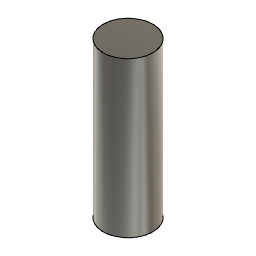
Lymphedema Project  Assembly v12 (Autodesk Fusion 360 archive; units mm, degrees)
design "Hand Model"
Autodesk Fusion 360 part; units mm, degrees
sketch "Sketch1" plane through (0, 0, 0) normal (0, 1, 0) x (1, 0, 0)
  circle A0 through (40, 0, 0) (-20, 0, 34.641) (-20, 0, -34.641)
  dimension "d1" = 80
extrude "Extrude1" add sketch "Sketch1" against normal blind 250 contours A0 in plane through (0, 0, 0) normal (0, 0, -1)

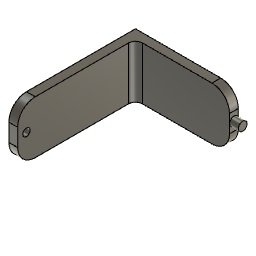
design "dummy wheel bracket"
Autodesk Fusion 360 part; units mm, degrees
sketch "Sketch1" plane through (0, 0, 0) normal (0, 0, 1) x (1, 0, 0)
  line L0 (-50, 0) -> (3.5, 0)
  line L1 (-50, 0) -> (-50, -67)
  line L2 (-50, -67) -> (-55, -67)
  line L3 (-55, -67) -> (-55, 5)
  line L4 (-55, 5) -> (3.5, 5)
  line L5 (3.5, 5) -> (3.5, 0)
  dimension "d1" = 53.5
  dimension "d2" = 67
  dimension "d3" = 5
  dimension "d8" = 5
  constraint horizontal L0
  constraint perpendicular L0 L1
  constraint perpendicular L1 L2
  constraint perpendicular L2 L3
  constraint perpendicular L3 L4
  measures "d1" distance of L0.start L0.end
  measures "d2" distance of L0.start L1.end
  measures "d3" distance of L1.end L2.end
  measures "d8" distance of L0.end L4.end
extrude "Extrude1" add sketch "Sketch1" along normal blind 30
sketch "Sketch2" plane through (3.5, 0, 0) normal (1, 0, 0) x (0, 1, 0)
  line L0 (0, 0) -> (5, 0)
  line L1 (5, 0) -> (5, 30)
  line L2 (5, 30) -> (0, 30)
  line L3 (0, 30) -> (0, 0)
  circle A0 centre (2.5, 15) radius 2.5
  dimension "d10" = 5
  measures "d10" diameter of A0
extrude "Extrude2" add sketch "Sketch2" along normal blind 5 contours A0
sketch "Sketch3" plane through (-50, 0, 0) normal (1, 0, 0) x (0, 1, 0)
  line L0 (-67, 0) -> (0, 0)
  line L1 (0, 0) -> (0, 30)
  line L2 (0, 30) -> (-67, 30)
  line L3 (-67, 30) -> (-67, 0)
  circle A0 centre (-62, 15) radius 2.1
  dimension "d14" = 4.2
  dimension "d17" = 5
  measures "d14" diameter of A0
  measures "d17" distance of L3 A0.centre
extrude "Extrude3" cut sketch "Sketch3" against normal blind 12 contours A0
fillet "Fillet1" radius 10 4 edges at (-52.5, -67, 30) (-52.5, -67, 0) (3.5, 2.5, 0) (3.5, 2.5, 30)
fillet "Fillet2" radius 4 1 edges at (-50, 0, 15)
equation "d1 = ( 117 / 2 ) * 1 mm - 5 mm"
equation "d2 = 100 mm - 33 mm"

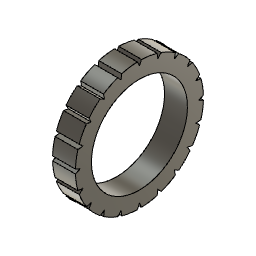
design "Soft Robotic Silicone Ring"
Autodesk Fusion 360 part; units mm, degrees
sketch "Sketch1" plane through (0, 0, 0) normal (0, 0, 1) x (1, 0, 0)
  line L0 (0, -42) -> (-10, -42)
  line L1 (-10, -42) -> (-10, -56)
  line L2 (-10, -56) -> (10, -56)
  line L3 (10, -56) -> (10, -42)
  line L4 (10, -42) -> (0, -42)
  dimension "d1" = 42
  dimension "d2" = 10
  dimension "d3" = 14
  dimension "d4" = 20
  dimension "d5" = 14
  constraint perpendicular L0 L1
  constraint perpendicular L1 L2
  constraint perpendicular L2 L3
  measures "d1" distance of origin L0.start
  measures "d2" distance of L0.start L0.end
  measures "d3" distance of L0.end L1.end
  measures "d4" distance of L1.end L2.end
  measures "d5" distance of L2.end L3.end
revolve "Revolve1" add sketch "Sketch1" angle 360 about axis through (1.75, 0, 0) along (1, 0, 0)
sketch "Sketch2" plane through (10, 0, 0) normal (1, 0, 0) x (0, 1, 0)
  circle A0 centre (0, 0) radius 42
  circle A1 centre (0, 0) radius 56
  line L0 (-52, 0) -> (-55.9694, -1.851)
  line L1 (-52, 0) -> (-55.9694, 1.851)
  arc A2 (-55.9694, 1.851) -> (-55.9694, -1.851) centre (0, 0) ccw
  line L2 (-49.4549, -16.0689) -> (-53.802, -15.5351)
  line L3 (-49.4549, -16.0689) -> (-52.6581, -19.0559)
  arc A3 (-53.802, -15.5351) -> (-52.6581, -19.0559) centre (0, 0) ccw
  line L4 (-42.0689, -30.5648) -> (-46.3682, -31.4005)
  line L5 (-42.0689, -30.5648) -> (-44.1922, -34.3954)
  arc A4 (-46.3682, -31.4005) -> (-44.1922, -34.3954) centre (0, 0) ccw
  line L6 (-30.5648, -42.0689) -> (-34.3954, -44.1922)
  line L7 (-30.5648, -42.0689) -> (-31.4005, -46.3682)
  arc A5 (-34.3954, -44.1922) -> (-31.4005, -46.3682) centre (0, 0) ccw
  line L8 (-16.0689, -49.4549) -> (-19.0559, -52.6581)
  line L9 (-16.0689, -49.4549) -> (-15.5351, -53.802)
  arc A6 (-19.0559, -52.6581) -> (-15.5351, -53.802) centre (0, 0) ccw
  line L10 (0, -52) -> (-1.851, -55.9694)
  line L11 (0, -52) -> (1.851, -55.9694)
  arc A7 (-1.851, -55.9694) -> (1.851, -55.9694) centre (0, 0) ccw
  line L12 (16.0689, -49.4549) -> (15.5351, -53.802)
  line L13 (16.0689, -49.4549) -> (19.0559, -52.6581)
  arc A8 (15.5351, -53.802) -> (19.0559, -52.6581) centre (0, 0) ccw
  line L14 (30.5648, -42.0689) -> (31.4005, -46.3682)
  line L15 (30.5648, -42.0689) -> (34.3954, -44.1922)
  arc A9 (31.4005, -46.3682) -> (34.3954, -44.1922) centre (0, 0) ccw
  line L16 (42.0689, -30.5648) -> (44.1922, -34.3954)
  line L17 (42.0689, -30.5648) -> (46.3682, -31.4005)
  arc A10 (44.1922, -34.3954) -> (46.3682, -31.4005) centre (0, 0) ccw
  line L18 (49.4549, -16.0689) -> (52.6581, -19.0559)
  line L19 (49.4549, -16.0689) -> (53.802, -15.5351)
  arc A11 (52.6581, -19.0559) -> (53.802, -15.5351) centre (0, 0) ccw
  line L20 (52, 0) -> (55.9694, -1.851)
  line L21 (52, 0) -> (55.9694, 1.851)
  arc A12 (55.9694, -1.851) -> (55.9694, 1.851) centre (0, 0) ccw
  line L22 (49.4549, 16.0689) -> (53.802, 15.5351)
  line L23 (49.4549, 16.0689) -> (52.6581, 19.0559)
  arc A13 (53.802, 15.5351) -> (52.6581, 19.0559) centre (0, 0) ccw
  line L24 (42.0689, 30.5648) -> (46.3682, 31.4005)
  line L25 (42.0689, 30.5648) -> (44.1922, 34.3954)
  arc A14 (46.3682, 31.4005) -> (44.1922, 34.3954) centre (0, 0) ccw
  line L26 (30.5648, 42.0689) -> (34.3954, 44.1922)
  line L27 (30.5648, 42.0689) -> (31.4005, 46.3682)
  arc A15 (34.3954, 44.1922) -> (31.4005, 46.3682) centre (0, 0) ccw
  line L28 (16.0689, 49.4549) -> (19.0559, 52.6581)
  line L29 (16.0689, 49.4549) -> (15.5351, 53.802)
  arc A16 (19.0559, 52.6581) -> (15.5351, 53.802) centre (0, 0) ccw
  line L30 (0, 52) -> (1.851, 55.9694)
  line L31 (0, 52) -> (-1.851, 55.9694)
  arc A17 (1.851, 55.9694) -> (-1.851, 55.9694) centre (0, 0) ccw
  line L32 (-16.0689, 49.4549) -> (-15.5351, 53.802)
  line L33 (-16.0689, 49.4549) -> (-19.0559, 52.6581)
  arc A18 (-15.5351, 53.802) -> (-19.0559, 52.6581) centre (0, 0) ccw
  line L34 (-30.5648, 42.0689) -> (-31.4005, 46.3682)
  line L35 (-30.5648, 42.0689) -> (-34.3954, 44.1922)
  arc A19 (-31.4005, 46.3682) -> (-34.3954, 44.1922) centre (0, 0) ccw
  line L36 (-42.0689, 30.5648) -> (-44.1922, 34.3954)
  line L37 (-42.0689, 30.5648) -> (-46.3682, 31.4005)
  arc A20 (-44.1922, 34.3954) -> (-46.3682, 31.4005) centre (0, 0) ccw
  line L38 (-49.4549, 16.0689) -> (-52.6581, 19.0559)
  line L39 (-49.4549, 16.0689) -> (-53.802, 15.5351)
  arc A21 (-52.6581, 19.0559) -> (-53.802, 15.5351) centre (0, 0) ccw
  point P0 (-56, 0)
  dimension "d7" = 4
  dimension "d11" = 360
  constraint coincident A1 L0.end
  constraint coincident A1 L1.end
  measures "d7" distance of P0 L0.start
extrude "Extrude1" cut sketch "Sketch2" against normal blind 50 contours A1 L20 L21 A12 | A1 L22 L23 A13 | A1 L18 L19 A11 | A1 L24 L25 A14 | A1 L16 L17 A10 | A1 L26 L27 A15 | A1 L14 L15 A9 | A1 L28 L29 A16 | A1 L12 L13 A8 | A1 L30 L31 A17 | A1 L10 L11 A7 | A1 L32 L33 A18 | A1 L8 L9 A6 | A1 L34 L35 A19 | A1 L6 L7 A5 | A1 L36 L37 A20 | A1 L4 L5 A4 | A1 L38 L39 A21 | A1 L2 L3 A3 | A1 L0 L1 A2
